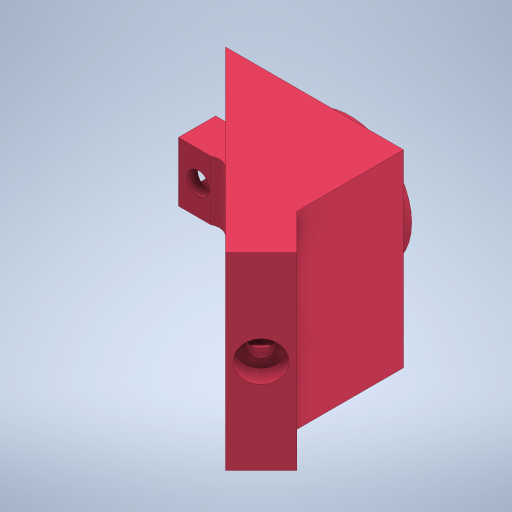
# Autodesk Inventor part: SpiegelSlider
Saved by Autodesk Inventor 2023 (Build 270158030, 158C)
## iProperties
Created: 2022-03-08
Part Number: SpiegelSlider
Material: Generic
Document SubType Name: Modeling
Designer: XFCM
Density: 1 g/cm^3
Appearance: Default
Author: XFCM
Autodesk Inventor part; units mm, degrees
ref_plane "YZ Plane" through (0, 0, 0) normal (1, 0, 0) x (0, 1, 0)
ref_plane "XZ Plane" through (0, 0, 0) normal (0, 1, 0) x (-1, 0, 0)
ref_plane "XY Plane" through (0, 0, 0) normal (0, 0, 1) x (1, 0, 0)
sketch "Sketch1" plane through (0, 0, 0) normal (0, 1, 0) x (-1, 0, 0)
  line L0 (0, 0) -> (35.921, -35.921)
  line L1 (0, 0) -> (50.8, 0) construction
  line L2 (0, 0) -> (0, -35.921)
  line L3 (0, -35.921) -> (35.921, -35.921)
  line L4 (0, 0) -> (-7.1842, -7.1842)
  line L5 (-7.1842, -7.1842) -> (0, -14.3684)
  point P0 (31.4309, -31.4309)
  dimension "d0" = 50.8
  dimension "d1" = 45
  dimension "d10" = 10.16
  constraints: 12 end point, 2 perpendicular, 2 point on line, 1 equal length, 1 horizontal, 1 vertical
  measures "d0" distance of L0.start L0.end
  measures "d1" angle of L0 L1
  measures "d10" distance of L0.start L4.end
extrude "Extrusion1" add sketch "Sketch1" along normal blind 38.1
sketch "Sketch2" plane through (0, 0, 0) normal (-0.7071068, 0, 0.7071068) x (0.7071068, 0, 0.7071068)
  line L0 (0, 0) -> (0, 38.1) projected
  line L1 (0, 0) -> (-25.4, 0)
  line L2 (-25.4, 0) -> (-25.4, 19.05)
  line L3 (-25.4, 19.05) -> (0, 19.05)
  line L4 (0, 19.05) -> (0, 0)
  circle A0 centre (-25.4, 19.05) radius 13.97
  line L5 (-11.43, 19.05) -> (-6.35, 19.05)
  line L6 (-6.35, 19.05) -> (-8.128, 19.05)
  line L7 (-8.128, 19.05) -> (-8.128, 23.114)
  line L8 (-8.128, 23.114) -> (-6.35, 23.114)
  line L9 (-6.35, 23.114) -> (-6.35, 19.05)
  line L10 (-6.35, 23.114) -> (-9.906, 23.114)
  line L11 (-9.906, 23.114) -> (-9.906, 14.986)
  line L12 (-9.906, 14.986) -> (-6.35, 14.986)
  line L13 (-6.35, 14.986) -> (-6.35, 23.114)
  dimension "d6" = 27.94
  dimension "d4" = 25.4
  dimension "d5" = 19.05
  dimension "d20" = 5.08
  dimension "d21" = 1.778
  dimension "d22" = 4.064
  dimension "d23" = 8.128
  constraints: 26 end point, 6 parallel, 3 horizontal, 3 perpendicular, 2 point on line, 1 coincident, 1 horizontal alignment, 2 other
  measures "d4" distance of L2.end L3.end
  measures "d5" distance of L1.end L2.end
  measures "d20" distance of L5.start L5.end
  measures "d21" distance of L7.end L8.end
  measures "d22" distance of L6.end L7.end
  measures "d23" distance of L11.end L10.end
extrude "Extrusion2" cut sketch "Sketch2" against normal blind 7.62 contours A0 L3 L2 | L2 L3 A0
sketch "Sketch3" plane through (7.1842, 0, -7.1842) normal (0.7071068, 0, 0.7071068) x (0.7071068, 0, -0.7071068)
  line L0 (-10.16, 0) -> (0, 0) projected
  line L1 (0, 0) -> (-5.08, 0)
  line L2 (-5.08, 0) -> (-5.08, 19.05)
  line L3 (-5.08, 19.05) -> (0, 19.05)
  line L4 (0, 19.05) -> (0, 0)
  dimension "d11" = 5.08
  dimension "d12" = 19.05
  constraints: 8 end point, 2 parallel, 1 horizontal, 1 perpendicular
  measures "d11" distance of L2.end L3.end
  measures "d12" distance of L1.end L2.end
hole "Hole1" at (3.5921, 19.05, -3.5921) direction (-0.7071068, 0, -0.7071068) diameter 4.4958 depth 12.7 tip angle 118 counterbore diameter 8.001 counterbore depth 3.9878 clearance for "Socket Head Cap Screw" size "M4" standard "Ansi Metric M Profile"
extrude "Extrusion3" cut sketch "Sketch2" against normal up to surface (10.16 mm away) contours L13 L12 L11 L3 | L3 L7 L8 L9 | L3 L11 L10 L7
sketch "Sketch4" plane through (0, 0, -35.921) normal (0, 0, -1) x (-1, 0, 0)
  circle A0 centre (17.9605, 19.05) radius 12.5
  line L0 (35.921, 38.1) -> (0, 38.1) projected
  line L1 (35.921, 38.1) -> (30.4605, 38.1)
  line L2 (30.4605, 38.1) -> (30.4605, 19.05)
  line L3 (30.4605, 19.05) -> (35.921, 19.05)
  line L4 (35.921, 19.05) -> (35.921, 38.1)
  line L5 (35.921, 19.05) -> (37.921, 19.05)
  line L6 (37.921, 19.05) -> (37.921, 22.05)
  line L7 (37.921, 22.05) -> (35.921, 22.05)
  line L8 (35.921, 22.05) -> (35.921, 19.05)
  line L9 (35.921, 0) -> (35.921, 38.1) projected
  line L10 (37.921, 22.05) -> (35.921, 22.05)
  line L11 (35.921, 22.05) -> (35.921, 16.05)
  line L12 (35.921, 16.05) -> (37.921, 16.05)
  line L13 (37.921, 16.05) -> (37.921, 22.05)
  line L14 (37.921, 22.05) -> (33.921, 22.05)
  line L15 (33.921, 22.05) -> (33.921, 19.05)
  line L16 (33.921, 19.05) -> (37.921, 19.05)
  line L17 (37.921, 19.05) -> (37.921, 22.05)
  line L18 (33.921, 19.05) -> (35.921, 19.05)
  line L19 (35.921, 19.05) -> (35.921, 16.05)
  line L20 (35.921, 16.05) -> (33.921, 16.05)
  line L21 (33.921, 16.05) -> (33.921, 19.05)
  line L22 (33.921, 22.05) -> (31.421, 22.05)
  line L23 (31.421, 22.05) -> (31.421, 16.05)
  line L24 (31.421, 16.05) -> (33.921, 16.05)
  line L25 (33.921, 16.05) -> (33.921, 22.05)
  line L26 (37.921, 22.05) -> (31.421, 22.05)
  line L27 (31.421, 22.05) -> (31.421, 25.05)
  line L28 (31.421, 25.05) -> (37.921, 25.05)
  line L29 (37.921, 25.05) -> (37.921, 22.05)
  line L30 (37.921, 16.05) -> (31.421, 16.05)
  line L31 (31.421, 16.05) -> (31.421, 13.05)
  line L32 (31.421, 13.05) -> (37.921, 13.05)
  line L33 (37.921, 13.05) -> (37.921, 16.05)
  point P0 (0, 0)
  dimension "d26" = 25
  dimension "d30" = 2
  dimension "d31" = 3
  dimension "d32" = 6
  dimension "d33" = 4
  dimension "d43" = 2.5
  dimension "d44" = 6
  dimension "d50" = 3
  dimension "d51" = 3
  constraints: 64 end point, 16 parallel, 8 horizontal, 8 perpendicular, 3 point on line, 1 coincident, 1 horizontal alignment, 2 other
  measures "d30" distance of L7.end L6.end
  measures "d31" distance of L6.end L5.end
  measures "d32" distance of L11.end L10.end
  measures "d33" distance of L16.end L15.end
  measures "d43" distance of L24.end L23.end
  measures "d44" distance of L23.end L22.end
  measures "d50" distance of L26.end L27.end
  measures "d51" distance of L31.end L30.end
extrude "Extrusion4" add sketch "Sketch4" along normal blind 7.112 contours A0
extrude "Extrusion5" add sketch "Sketch4" against normal blind 7.5 contours L23 L22 L15 L3 | L3 L21 L24 L23 | L15 L14 L4 L3 | L3 L9 L20 L21 | L27 L28 L4 L14 L22 | L24 L20 L9 L32 L31 | L28 L29 L7 L4 | L4 L7 L6 L5 | L5 L13 L12 L9 | L12 L33 L32 L9
hole "Hole2" at (-33.921, 19.05, -35.921) direction (0, 0, 1) diameter 4.5 end through all clearance for "Flat Head Machine Screw" size "M4" standard "Ansi Metric M Profile"
fillet "Fillet1" radius 3 1 edges at (-31.421, 19.05, -31.421)
sketch "Sketch6" plane through (-37.921, 13.05, -35.921) normal (-1, 0, 0) x (0, 0, 1)
  line L0 (4.5, 3) -> (0, 0)
  line L1 (4.5, 3) -> (0, 3)
  line L2 (0, 3) -> (0, 2)
  line L3 (0, 2) -> (4.5, 2)
  line L4 (4.5, 2) -> (4.5, 3)
  line L5 (0, 2) -> (2, 2)
  line L6 (2, 2) -> (5.4, 2)
  line L7 (5.4, 2) -> (5.4, 10)
  line L8 (5.4, 10) -> (2, 10)
  line L9 (2, 10) -> (2, 2)
  line L10 (0, 0) -> (7.5, 0) projected
  point P0 (35.921, -13.05)
  point P1 (35.921, -16.05)
  point P2 (4.5, 2)
  dimension "d53" = 4.5
  dimension "d54" = 1
  dimension "d55" = 2
  dimension "d56" = 3.4
  dimension "d57" = 8
  dimension "d58" = 2
  constraints: 20 end point, 4 parallel, 2 horizontal, 2 perpendicular, 1 point on line
  measures "d53" distance of L3.end L2.end
  measures "d54" distance of L2.end L1.end
  measures "d55" distance of L2.end L5.end
  measures "d56" distance of L8.end L7.end
  measures "d57" distance of L7.end L6.end
  measures "d58" distance between parallel lines of L10 L6
extrude "Extrusion6" cut sketch "Sketch6" against normal blind 8 contours L4 L3 L0 | L0 L3 L9 L1 | L1 L9 L8 L7 L6 L4
draft "Flächenverjüngung1" angle 10 pull direction (0, 0, 1) faces at (-29.6901, 23.3705, -40.6624) fixed edges at (-5.4605, 19.05, -43.033)
body "Solid1"
